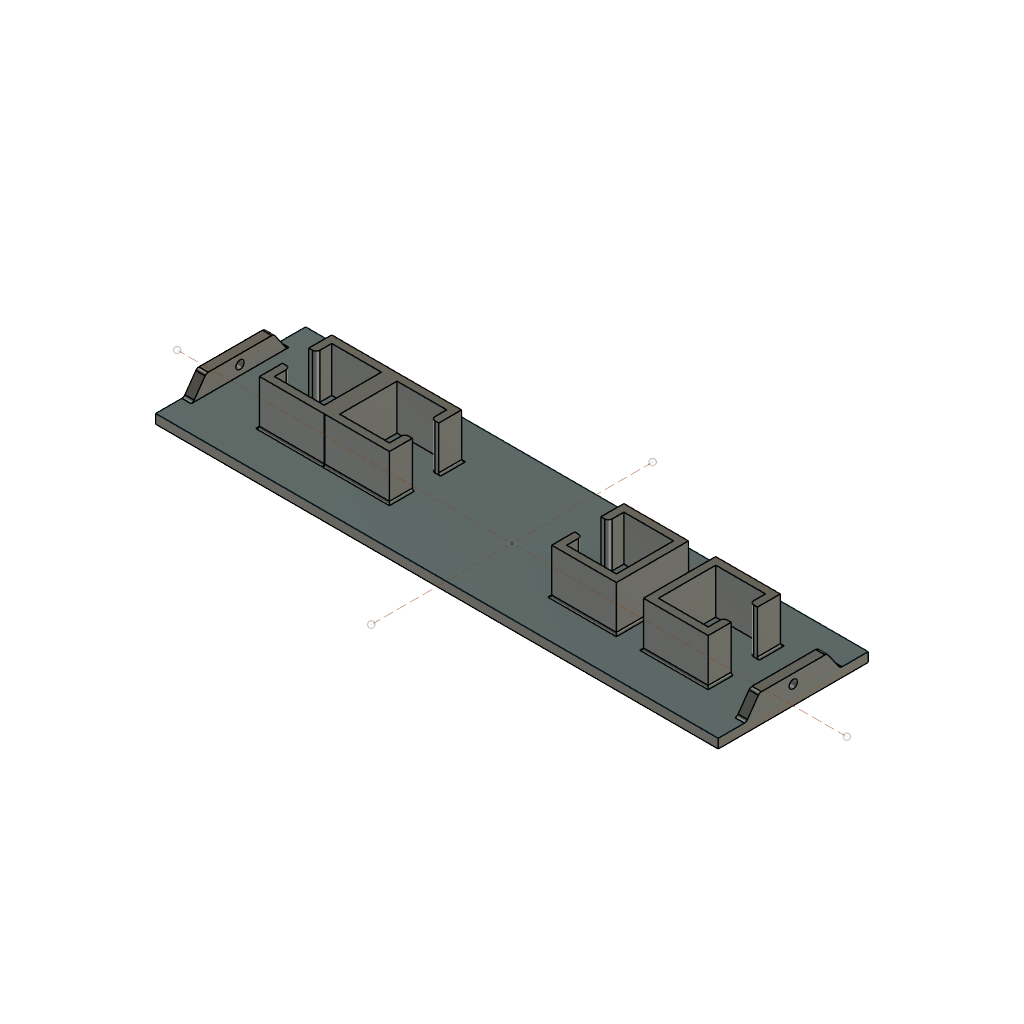
Actuator Plate (Autodesk Fusion 360 design; units mm, degrees)
part number: 2026-09-11-18-50-23-005
Autodesk Fusion 360 part; units mm, degrees
sketch "Sketch1" plane through (0, 0, 0) normal (0, 0, 1) x (1, 0, 0)
  line L0 (68.541, -12.5) -> (-110, -12.5) construction
  line L1 (-20.75, -50) -> (-20.75, 25) construction
  point P0 (-20.75, -12.5)
  constraint horizontal L0
  constraint midpoint L1 P0
  constraint coincident L0 P0
  constraint perpendicular L0 L1
sketch "Sketch2" plane through (0, 0, 0) normal (0, 0, 1) x (1, 0, 0)
  line L0 (54.25, 7.5) -> (-95.75, 7.5)
  line L1 (-95.75, 7.5) -> (-95.75, -32.5)
  line L2 (-95.75, -32.5) -> (54.25, -32.5)
  line L3 (54.25, -32.5) -> (54.25, 7.5)
  line L4 (54.25, 7.5) -> (-95.75, -32.5) construction
  line L5 (-95.75, 7.5) -> (54.25, -32.5) construction
  line L6 (26.6666, -12.5) -> (38.5, -12.5) construction
  circle A0 centre (32.5833, -12.5) radius 2.75
  line L7 (14, -12.5) -> (2.2, -12.5) construction
  circle A1 centre (8.1, -12.5) radius 2.75
  line L8 (-49.1, -12.5) -> (-52.4, -12.5) construction
  circle A2 centre (-52.4, -12.5) radius 2.75
  line L9 (-73.1, -12.5) -> (-69.8, -12.5) construction
  circle A3 centre (-69.8, -12.5) radius 2.75
  point P0 (-20.75, -12.5)
  dimension "d1" = 150
  dimension "d2" = 40
  dimension "d3" = 5.5
  dimension "d4" = 5.5
  dimension "d5" = 3.3
  dimension "d6" = 5.5
  dimension "d7" = 3.3
  dimension "d8" = 5.5
  constraint horizontal L0
  constraint perpendicular L0 L1
  constraint parallel L0 L2
  constraint parallel L1 L3
  constraint coincident L4 P0
  constraint coincident L5 P0
  constraint horizontal L6
  constraint midpoint L6 A0.centre
  constraint horizontal L7
  constraint midpoint L7 A1.centre
  constraint horizontal L8
  constraint coincident L8.end A2.centre
  constraint horizontal L9
  constraint coincident L9.end A3.centre
  measures "d1" distance of L1.end L2.end
  measures "d2" distance of L0.end L1.end
  measures "d3" diameter of A0
  measures "d4" diameter of A1
  measures "d5" distance of L8.start L8.end
  measures "d6" diameter of A2
  measures "d7" distance of L9.start L9.end
  measures "d8" diameter of A3
extrude "Extrude1" add sketch "Sketch2" along normal blind 2.5
sketch "Sketch3" plane through (0, 0, 2.5) normal (0, 0, 1) x (-1, 0, 0)
  circle A0 centre (-32.5833, 12.5) radius 2.75
  circle A1 centre (69.8, 12.5) radius 2.75
  circle A2 centre (-8.1, 12.5) radius 2.75
  circle A3 centre (52.4, 12.5) radius 2.75
  line L0 (-54.25, 32.5) -> (-54.25, -7.5)
  line L1 (-54.25, -7.5) -> (95.75, -7.5)
  line L2 (95.75, -7.5) -> (95.75, 32.5)
  line L3 (95.75, 32.5) -> (-54.25, 32.5)
sketch "Sketch4" plane through (0, 0, 2.5) normal (0, 0, 1) x (-1, 0, 0)
  line L0 (-29.8338, 12.5) -> (-35.3337, 12.5) construction
  line L1 (-39.2087, 4.875) -> (-25.9587, 4.875)
  line L2 (-25.9587, 4.875) -> (-25.9587, 20.125)
  line L3 (-25.9587, 20.125) -> (-39.2087, 20.125)
  line L4 (-39.2087, 20.125) -> (-39.2087, 4.875)
  line L5 (-39.2087, 4.875) -> (-25.9587, 20.125) construction
  line L6 (-25.9587, 4.875) -> (-39.2087, 20.125) construction
  line L7 (-41.2087, 2.875) -> (-23.9587, 2.875)
  line L8 (-23.9587, 2.875) -> (-23.9587, 22.125)
  line L9 (-23.9587, 22.125) -> (-41.2087, 22.125)
  line L10 (-41.2087, 22.125) -> (-41.2087, 2.875)
  line L11 (-41.2087, 2.875) -> (-23.9587, 22.125) construction
  line L12 (-23.9587, 2.875) -> (-41.2087, 22.125) construction
  line L13 (-39.2087, 12.5) -> (-39.2087, 9)
  line L14 (-39.2087, 9) -> (-41.2087, 9)
  line L15 (-41.2087, 9) -> (-41.2087, 16)
  line L16 (-41.2087, 16) -> (-39.2087, 16)
  line L17 (-39.2087, 16) -> (-39.2087, 12.5)
  line L18 (-5.35, 12.5) -> (-10.85, 12.5) construction
  line L19 (-14.725, 4.875) -> (-1.475, 4.875)
  line L20 (-1.475, 4.875) -> (-1.475, 20.125)
  line L21 (-1.475, 20.125) -> (-14.725, 20.125)
  line L22 (-14.725, 20.125) -> (-14.725, 4.875)
  line L23 (-14.725, 4.875) -> (-1.475, 20.125) construction
  line L24 (-1.475, 4.875) -> (-14.725, 20.125) construction
  line L25 (-16.725, 2.875) -> (0.525, 2.875)
  line L26 (0.525, 2.875) -> (0.525, 22.125)
  line L27 (0.525, 22.125) -> (-16.725, 22.125)
  line L28 (-16.725, 22.125) -> (-16.725, 2.875)
  line L29 (-16.725, 2.875) -> (0.525, 22.125) construction
  line L30 (0.525, 2.875) -> (-16.725, 22.125) construction
  line L31 (-1.475, 16) -> (-1.475, 9)
  line L32 (0.525, 16) -> (0.525, 9)
  line L33 (0.525, 9) -> (-1.475, 9)
  line L34 (0.525, 16) -> (-1.475, 16)
  line L35 (55.15, 12.5) -> (49.65, 12.5) construction
  line L36 (45.775, 4.875) -> (59.025, 4.875)
  line L37 (59.025, 4.875) -> (59.025, 20.125)
  line L38 (59.025, 20.125) -> (45.775, 20.125)
  line L39 (45.775, 20.125) -> (45.775, 4.875)
  line L40 (45.775, 4.875) -> (59.025, 20.125) construction
  line L41 (59.025, 4.875) -> (45.775, 20.125) construction
  line L42 (61.025, 22.125) -> (43.775, 22.125)
  line L43 (43.775, 22.125) -> (43.775, 2.875)
  line L44 (43.775, 2.875) -> (61.025, 2.875)
  line L45 (61.025, 22.125) -> (43.775, 2.875) construction
  line L46 (43.775, 22.125) -> (61.025, 2.875) construction
  line L47 (72.55, 12.5) -> (67.05, 12.5) construction
  line L48 (63.175, 4.875) -> (76.425, 4.875)
  line L49 (76.425, 4.875) -> (76.425, 20.125)
  line L50 (76.425, 20.125) -> (63.175, 20.125)
  line L51 (63.175, 20.125) -> (63.175, 4.875)
  line L52 (63.175, 4.875) -> (76.425, 20.125) construction
  line L53 (76.425, 4.875) -> (63.175, 20.125) construction
  line L54 (61.175, 2.875) -> (78.425, 2.875)
  line L55 (78.425, 2.875) -> (78.425, 22.125)
  line L56 (78.425, 22.125) -> (61.175, 22.125)
  line L57 (61.175, 2.875) -> (78.425, 22.125) construction
  line L58 (78.425, 2.875) -> (61.175, 22.125) construction
  line L59 (61.175, 2.875) -> (61.025, 2.875)
  line L60 (61.175, 22.125) -> (61.025, 22.125)
  line L61 (43.775, 16) -> (43.775, 9)
  line L62 (45.775, 16) -> (45.775, 9)
  line L63 (45.775, 9) -> (43.775, 9)
  line L64 (45.775, 16) -> (43.775, 16)
  line L65 (76.425, 16) -> (76.425, 9)
  line L66 (78.425, 16) -> (78.425, 9)
  line L67 (78.425, 9) -> (76.425, 9)
  line L68 (76.425, 16) -> (78.425, 16)
  point P0 (-32.5837, 12.5)
  point P1 (-32.5837, 12.5)
  point P2 (-8.1, 12.5)
  point P3 (-8.1, 12.5)
  point P4 (-1.475, 12.5)
  point P5 (0.525, 12.5)
  point P6 (52.4, 12.5)
  point P7 (52.4, 12.5)
  point P8 (69.8, 12.5)
  point P9 (69.8, 12.5)
  point P10 (43.775, 12.5)
  point P11 (45.775, 12.5)
  point P12 (76.425, 12.5)
  point P13 (78.425, 12.5)
  dimension "d11" = 13.25
  dimension "d12" = 15.25
  dimension "d13" = 17.25
  dimension "d14" = 19.25
  dimension "d15" = 3.5
  dimension "d16" = 7
  dimension "d17" = 13.25
  dimension "d18" = 15.25
  dimension "d19" = 17.25
  dimension "d20" = 19.25
  dimension "d21" = 7
  dimension "d22" = 7
  dimension "d23" = 13.25
  dimension "d24" = 15.25
  dimension "d25" = 17.25
  dimension "d26" = 19.25
  dimension "d27" = 13.25
  dimension "d28" = 15.25
  dimension "d29" = 17.25
  dimension "d30" = 19.25
  dimension "d31" = 7
  dimension "d32" = 7
  dimension "d33" = 7
  dimension "d34" = 7
  constraint horizontal L0
  constraint horizontal L1
  constraint perpendicular L1 L2
  constraint parallel L1 L3
  constraint parallel L2 L4
  constraint coincident L5 P1
  constraint coincident L6 P1
  constraint midpoint L0 P1
  constraint horizontal L7
  constraint perpendicular L7 L8
  constraint parallel L7 L9
  constraint parallel L8 L10
  constraint coincident L11 P1
  constraint coincident L12 P1
  constraint coincident P1 P0
  constraint midpoint L4 L13.start
  constraint coincident L4 L13.end
  constraint coincident L10 L14.end
  constraint perpendicular L10 L14
  constraint perpendicular L14 L15
  constraint coincident L4 L16.end
  constraint perpendicular L4 L16
  constraint horizontal L18
  constraint horizontal L19
  constraint perpendicular L19 L20
  constraint parallel L19 L21
  constraint parallel L20 L22
  constraint coincident L23 P3
  constraint coincident L24 P3
  constraint midpoint L18 P3
  constraint horizontal L25
  constraint perpendicular L25 L26
  constraint parallel L25 L27
  constraint parallel L26 L28
  constraint coincident L29 P3
  constraint coincident L30 P3
  constraint coincident P3 P2
  constraint midpoint L31 P4
  constraint coincident L20 P4
  constraint parallel L20 L31
  constraint midpoint L32 P5
  constraint coincident L26 P5
  constraint parallel L26 L32
  constraint perpendicular L20 L33
  constraint horizontal L35
  constraint horizontal L36
  constraint perpendicular L36 L37
  constraint parallel L36 L38
  constraint parallel L37 L39
  constraint coincident L40 P7
  constraint coincident L41 P7
  constraint midpoint L35 P7
  constraint horizontal L42
  constraint perpendicular L42 L43
  constraint parallel L42 L44
  constraint coincident L45 P7
  constraint coincident L46 P7
  constraint coincident P7 P6
  constraint perpendicular L37 L47
  constraint horizontal L48
  constraint perpendicular L48 L49
  constraint parallel L48 L50
  constraint parallel L49 L51
  constraint coincident L52 P9
  constraint coincident L53 P9
  constraint midpoint L47 P9
  constraint horizontal L54
  constraint perpendicular L54 L55
  constraint parallel L54 L56
  constraint coincident L57 P9
  constraint coincident L58 P9
  constraint coincident P9 P8
  constraint midpoint L61 P10
  constraint coincident L43 P10
  constraint parallel L43 L61
  constraint midpoint L62 P11
  constraint coincident L39 P11
  constraint parallel L39 L62
  constraint perpendicular L43 L63
  constraint midpoint L65 P12
  constraint coincident L49 P12
  constraint parallel L49 L65
  constraint midpoint L66 P13
  constraint coincident L55 P13
  constraint parallel L55 L66
  constraint perpendicular L49 L67
  measures "d11" distance of L2.end L3.end
  measures "d12" distance of L1.end L2.end
  measures "d13" distance of L8.end L9.end
  measures "d14" distance of L7.end L8.end
  measures "d15" distance of L13.start L13.end
  measures "d16" distance of L14.end L15.end
  measures "d17" distance of L20.end L21.end
  measures "d18" distance of L19.end L20.end
  measures "d19" distance of L26.end L27.end
  measures "d20" distance of L25.end L26.end
  measures "d21" distance of L31.start L31.end
  measures "d22" distance of L32.start L32.end
  measures "d23" distance of L37.end L38.end
  measures "d24" distance of L36.end L37.end
  measures "d25" distance of L43.end L44.end
  measures "d26" distance of L42.end L43.end
  measures "d27" distance of L49.end L50.end
  measures "d28" distance of L48.end L49.end
  measures "d29" distance of L55.end L56.end
  measures "d30" distance of L54.end L55.end
  measures "d31" distance of L61.start L61.end
  measures "d32" distance of L62.start L62.end
  measures "d33" distance of L65.start L65.end
  measures "d34" distance of L66.start L66.end
extrude "Extrude2" add sketch "Sketch4" along normal blind 12 contours L1 L2 L3 L4 L7 L8 L9 L10 L14 L16 | L19 L20 L21 L22 L25 L26 L27 L28 L33 L34 | L36 L37 L38 L39 L42 L43 L44 L48 L49 L50 L51 L54 L55 L56 L59 L60 L63 L64 L67 L68
sketch "Sketch5" plane through (0, 0, 2.5) normal (0, 0, 1) x (-1, 0, 0)
sketch "Sketch7" plane through (54.25, 0, 0) normal (1, 0, 0) x (0, 1, 0)
  line L0 (-32.5, 0) -> (7.5, 0)
  line L1 (7.5, 0) -> (7.5, 2.5)
  line L2 (7.5, 2.5) -> (-32.5, 2.5)
  line L3 (-32.5, 2.5) -> (-32.5, 0)
  line L4 (-25, 2.5) -> (0, 2.5)
  line L5 (-21.5, 2.5) -> (-3.5, 2.5)
  line L6 (-12.5, 7.5) -> (-3.5, 7.5)
  line L7 (-3.5, 7.5) -> (0, 2.5)
  line L8 (-12.5, 7.5) -> (-21.5, 7.5)
  line L9 (-21.5, 7.5) -> (-25, 2.5)
  line L10 (-12.5, 2.5) -> (-12.5, 7.5) construction
  circle A0 centre (-12.5, 5) radius 1.1
  point P0 (-12.5, 2.5)
  point P1 (-12.5, 2.5)
  dimension "d39" = 25
  dimension "d40" = 18
  dimension "d41" = 2.2
  constraint midpoint L4 P1
  constraint coincident L2 P1
  constraint parallel L2 L4
  constraint midpoint L5 P1
  constraint coincident P1 P0
  constraint parallel L4 L5
  constraint perpendicular L8 L10
  constraint midpoint L10 A0.centre
  measures "d39" distance of L4.start L4.end
  measures "d40" distance of L5.start L5.end
  measures "d41" diameter of A0
extrude "Extrude3" add sketch "Sketch7" against normal blind 2.5 contours L2 L4 L5 L6 L7 L8 L9
sketch "Sketch8" plane through (-95.75, 0, 0) normal (-1, 0, 0) x (0, -1, 0)
  line L0 (-7.5, 0) -> (32.5, 0)
  line L1 (32.5, 0) -> (32.5, 2.5)
  line L2 (32.5, 2.5) -> (-7.5, 2.5)
  line L3 (-7.5, 2.5) -> (-7.5, 0)
  line L4 (0, 2.5) -> (25, 2.5)
  line L5 (3.5, 7.5) -> (21.5, 7.5)
  line L6 (3.5, 7.5) -> (0, 2.5)
  line L7 (21.5, 7.5) -> (25, 2.5)
  circle A0 centre (12.5, 5) radius 1.1
  point P0 (12.5, 2.5)
  dimension "d44" = 25
  dimension "d46" = 18
  dimension "d47" = 2.2
  constraint midpoint L4 P0
  constraint coincident L2 P0
  constraint parallel L2 L4
  measures "d44" distance of L4.start L4.end
  measures "d46" distance of L5.start L5.end
  measures "d47" diameter of A0
extrude "Extrude4" add sketch "Sketch8" against normal blind 2.5 contours L2 L4 L5 L6 L7
fillet "Fillet1" radius 1 4 edges at (-94.5, -21.5, 7.5) (-94.5, -25, 2.5) (-94.5, -3.5, 7.5) (-94.5, 0, 2.5)
fillet "Fillet2" radius 1 4 edges at (53, -25, 2.5) (53, -21.5, 7.5) (53, -3.5, 7.5) (53, 0, 2.5)
fillet "Fillet3" radius 0.5 5 edges at (41.2087, -19.0625, 2.5) (32.5837, -22.125, 2.5) (41.2087, -5.9375, 2.5) (32.5837, -2.875, 2.5) (23.9587, -12.5, 2.5)
fillet "Fillet4" radius 0.5 15 edges at (16.725, -12.5, 2.5) (8.1, -2.875, 2.5) (8.1, -22.125, 2.5) (-0.525, -5.9375, 2.5) (-0.525, -19.0625, 2.5) (-52.4, -22.125, 2.5) (-61.1, -22.125, 2.5) (-69.8, -22.125, 2.5) (-78.425, -19.0625, 2.5) (-78.425, -5.9375, 2.5) (-43.775, -19.0625, 2.5) (-43.775, -5.9375, 2.5) (-69.8, -2.875, 2.5) (-61.1, -2.875, 2.5) (-52.4, -2.875, 2.5)
fillet "Fillet5" radius 1 8 edges at (-45.775, -16, 8.5) (-45.775, -9, 8.5) (-76.425, -9, 8.5) (-76.425, -16, 8.5) (1.475, -16, 8.5) (1.475, -9, 8.5) (39.2087, -16, 8.5) (39.2087, -9, 8.5)
